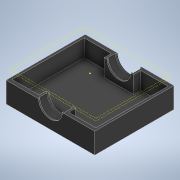
# Autodesk Inventor part: caja_base
Saved by Autodesk Inventor 2021 (Build 250183000, 183)
## iProperties
Created: 2021-12-11
Part Number: caja_base
Material: Generic
Document SubType Name: Modeling
Designer: Juan M. Casillas
Density: 1 g/cm^3
Appearance: Default
Author: Juan M. Casillas
Autodesk Inventor part; units mm, degrees
ref_plane "YZ Plane" through (0, 0, 0) normal (1, 0, 0) x (0, 1, 0)
ref_plane "XZ Plane" through (0, 0, 0) normal (0, 1, 0) x (-1, 0, 0)
ref_plane "XY Plane" through (0, 0, 0) normal (0, 0, 1) x (1, 0, 0)
sketch "Sketch1" plane through (0, 0, 0) normal (0, 1, 0) x (-1, 0, 0)
  line L0 (37.5, 32.5) -> (-37.5, 32.5)
  line L1 (-37.5, 32.5) -> (-37.5, -32.5)
  line L2 (-37.5, -32.5) -> (37.5, -32.5)
  line L3 (37.5, -32.5) -> (37.5, 32.5)
  line L4 (37.5, 32.5) -> (-37.5, -32.5) construction
  line L5 (-37.5, 32.5) -> (37.5, -32.5) construction
  line L6 (35.5, 30.5) -> (-35.5, 30.5)
  line L7 (-35.5, 30.5) -> (-35.5, -30.5)
  line L8 (-35.5, -30.5) -> (35.5, -30.5)
  line L9 (35.5, -30.5) -> (35.5, 30.5)
  line L10 (-12.5, -30.5) -> (12.5, -30.5)
  line L11 (12.5, -30.5) -> (12.5, -23.5)
  line L12 (12.5, -23.5) -> (-12.5, -23.5)
  line L13 (-12.5, -23.5) -> (-12.5, -30.5)
  line L14 (-12.5, 23.5) -> (12.5, 23.5)
  line L15 (12.5, 23.5) -> (12.5, 30.5)
  line L16 (12.5, 30.5) -> (-12.5, 30.5)
  line L17 (-12.5, 30.5) -> (-12.5, 23.5)
  point P0 (0, 0)
  point P1 (0, -30.5)
  point P2 (0, 30.5)
  point P3 (-12.5, -30.5)
  point P4 (12.5, -30.5)
  dimension "d0" = 75
  dimension "d1" = 65
  dimension "d2" = 2
  dimension "d7" = 25
  dimension "d8" = 7
  dimension "d9" = 25
  dimension "d10" = 7
  constraints: 36 end point, 8 parallel, 6 midpoint, 4 perpendicular, 3 horizontal, 3 other
  measures "d0" distance of L2.end L1.end
  measures "d1" distance of L1.end L0.end
  measures "d2" distance between parallel lines of L3 L9
  measures "d7" distance of L12.end L11.end
  measures "d8" distance of L11.end L10.end
  measures "d9" distance of L16.end L15.end
  measures "d10" distance of L15.end L14.end
extrude "Extrusion1" add sketch "Sketch1" along normal blind 20
sketch "Sketch2" plane through (0, 20, 0) normal (0, 1, 0) x (1, 0, 0)
  line L0 (-37.5, -32.5) -> (37.5, -32.5) construction
  line L1 (37.5, -32.5) -> (37.5, 32.5) construction
  line L2 (37.5, 32.5) -> (-37.5, 32.5) construction
  line L3 (-37.5, 32.5) -> (-37.5, -32.5) construction
  line L4 (-37.5, -32.5) -> (37.5, -32.5) construction
  line L5 (-35.5, -30.5) -> (-35.5, 30.5) construction
  line L6 (-35.5, 30.5) -> (35.5, 30.5) construction
  line L7 (35.5, 30.5) -> (35.5, -30.5) construction
  line L8 (35.5, -30.5) -> (-35.5, -30.5) construction
  point P0 (0, 0)
sketch "Sketch3" plane through (0, 0, 0) normal (0, -1, 0) x (1, 0, 0)
  line L0 (-37.5, 32.5) -> (37.5, 32.5) projected
  line L1 (37.5, 32.5) -> (37.5, -32.5) projected
  line L2 (37.5, -32.5) -> (-37.5, -32.5) projected
  line L3 (-37.5, -32.5) -> (-37.5, 32.5) projected
  point P0 (0, 0)
extrude "Extrusion2" add sketch "Sketch3" against normal blind 3
extrude "Extrusion3" add sketch "Sketch1" along normal blind 13 contours L15 L14 L17 L6 | L8 L13 L12 L11
sketch "Sketch4" plane through (-12.5, 3, -23.5) normal (0, 0, 1) x (1, 0, 0)
  line L0 (0, 10) -> (25, 10) construction
  point P0 (12.5, -3)
  point P1 (12.5, 10)
  constraints: 1 midpoint
hole "Hole2" at (0, 13, -23.5) direction (0, 0, -1) diameter 22 end through all both
thicken "Thicken1" operation add thickness 7 both sides no extend neighbours yes toward (0, -1, 0) faces at (36.8333, 20, 10.1667)
thicken "Thicken2" operation add thickness 7 both sides no extend neighbours yes toward (0, -1, 0) faces at (-36.8333, 20, 10.1667)
thicken "Thicken3" operation add thickness 1 both sides no extend neighbours yes toward (0, 0, 1) faces at (11.9049, 8.8371, 23.5)
thicken "Thicken4" operation add thickness 1 both sides no extend neighbours yes toward (0, 0, 1) faces at (-11.9049, 8.8371, 23.5)
thicken "Thicken5" operation add thickness 1 both sides no extend neighbours yes toward (0, 0, -1) faces at (11.9049, 8.8371, -23.5)
thicken "Thicken6" operation add thickness 1 both sides no extend neighbours yes toward (0, 0, -1) faces at (-11.9049, 8.8371, -23.5)
sketch "Sketch5" plane through (12.5, 3, 24.5) normal (0, 0, -1) x (-1, 0, 0)
  arc A0 (1.5, 10) -> (7.9174, 0) centre (12.5, 10) ccw projected
  arc A1 (17.0826, 0) -> (23.5, 10) centre (12.5, 10) ccw projected
  arc A2 (1.5, 10) -> (23.5, 10) centre (12.5, 10) ccw projected
  line L0 (1.5, 10) -> (2.5, 10)
  line L1 (23.5, 10) -> (22.5, 10)
  arc A3 (2.5, 10) -> (22.5, 10) centre (12.5, 10) ccw
  point P0 (12.5, -3)
  dimension "d39" = 1
  dimension "d40" = 1
  constraints: 4 end point, 2 horizontal, 2 point on circle, 1 centre point
  measures "d39" distance of L0.start L0.end
  measures "d40" distance of L1.start L1.end
extrude "Extrusion4" add sketch "Sketch5" against normal blind 1
thicken "Thicken7" operation add thickness 1 both sides no extend neighbours yes toward (0, 0, -1) faces at (11.5698, 8.8689, 24.5)
mirror "Mirror1" about plane through (0, 0, 0) normal (0, 0, 1) of "Extrusion4"
thicken "Thicken8" operation add thickness 1 both sides no extend neighbours yes toward (0, 0, 1) faces at (-11.5698, 8.8689, -24.5)
sketch "Sketch6" plane through (37.5, 0, -32.5) normal (0, 0, -1) x (-1, 0, 0)
  arc A0 (26.5, 13) -> (48.5, 13) centre (37.5, 13) ccw projected
  line L0 (47.5, 13) -> (48.5, 13) projected
  arc A1 (27.5, 13) -> (47.5, 13) centre (37.5, 13) ccw projected
  line L1 (26.5, 13) -> (27.5, 13) projected
  arc A2 (26.5, 13) -> (48.5, 13) centre (37.5, 13) ccw projected
  line L2 (0, 13) -> (26.5, 13) projected
  line L3 (0, 0) -> (0, 13) projected
  line L4 (0, 0) -> (75, 0) projected
  line L5 (75, 0) -> (75, 13) projected
  line L6 (48.5, 13) -> (75, 13) projected
  point P0 (37.5, 0)
extrude "Extrusion5" add sketch "Sketch6" along normal blind 1
mirror "Mirror2" about plane through (0, 0, 0) normal (0, 0, 1) of "Extrusion5"
thicken "Thicken9" operation add thickness 1 both sides no extend neighbours yes toward (0, 0, -1) faces at (-11.5698, 8.8689, -23.5)
thicken "Thicken10" operation add thickness 1 both sides no extend neighbours yes toward (0, 0, 1) faces at (11.5698, 8.8689, 23.5)
sketch "Sketch8" plane through (0, 0, 0) normal (0, -1, 0) x (1, 0, 0)
  line L0 (37.5, 33.5) -> (37.5, -33.5) projected
  line L1 (37.5, 33.5) -> (-37.5, 33.5) projected
  line L2 (-37.5, 33.5) -> (-37.5, -33.5) projected
  line L3 (37.5, -33.5) -> (-37.5, -33.5) projected
  point P0 (0, 0)
extrude "Extrusion6" add sketch "Sketch8" along normal blind 5
sketch "Sketch9" plane through (0, 3, 0) normal (0, 1, 0) x (1, 0, 0)
  line L0 (-4.5826, -24.5) -> (-4.5826, 24.5) projected
  line L1 (-4.5826, 24.5) -> (-12.5, 24.5) projected
  line L2 (-12.5, 24.5) -> (-12.5, 30.5) projected
  line L3 (-35.5, 30.5) -> (-12.5, 30.5) projected
  line L4 (-35.5, -30.5) -> (-35.5, 30.5) projected
  line L5 (-12.5, -30.5) -> (-35.5, -30.5) projected
  line L6 (-12.5, -30.5) -> (-12.5, -24.5) projected
  line L7 (-12.5, -24.5) -> (-4.5826, -24.5) projected
  line L8 (4.5826, 24.5) -> (-4.5826, 24.5) projected
  line L9 (-4.5826, -24.5) -> (-4.5826, 24.5) projected
  line L10 (-4.5826, -24.5) -> (4.5826, -24.5) projected
  line L11 (4.5826, 24.5) -> (4.5826, -24.5) projected
  line L12 (4.5826, 24.5) -> (4.5826, -24.5) projected
  line L13 (4.5826, -24.5) -> (12.5, -24.5) projected
  line L14 (12.5, -24.5) -> (12.5, -30.5) projected
  line L15 (35.5, -30.5) -> (12.5, -30.5) projected
  line L16 (35.5, 30.5) -> (35.5, -30.5) projected
  line L17 (12.5, 30.5) -> (35.5, 30.5) projected
  line L18 (12.5, 30.5) -> (12.5, 24.5) projected
  line L19 (12.5, 24.5) -> (4.5826, 24.5) projected
  line L20 (4.5826, 24.5) -> (4.5826, -24.5) projected
  line L21 (4.5826, -24.5) -> (12.5, -24.5) projected
  line L22 (12.5, -24.5) -> (12.5, -30.5) projected
  line L23 (35.5, -30.5) -> (12.5, -30.5) projected
  line L24 (35.5, 30.5) -> (35.5, -30.5) projected
  line L25 (12.5, 30.5) -> (35.5, 30.5) projected
  line L26 (12.5, 30.5) -> (12.5, 24.5) projected
  line L27 (12.5, 24.5) -> (4.5826, 24.5) projected
  point P0 (0, 0)
extrude "Extrusion7" cut sketch "Sketch9" against normal blind 5
sketch "Sketch10" plane through (0, -2, 0) normal (0, 1, 0) x (1, 0, 0)
  line L0 (12.5, -24.5) -> (-12.5, -24.5) projected
  line L1 (12.5, -30.5) -> (12.5, -24.5) projected
  line L2 (35.5, -30.5) -> (12.5, -30.5) projected
  line L3 (35.5, 30.5) -> (35.5, -30.5) projected
  line L4 (12.5, 30.5) -> (35.5, 30.5) projected
  line L5 (12.5, 24.5) -> (12.5, 30.5) projected
  line L6 (-12.5, 24.5) -> (12.5, 24.5) projected
  line L7 (-12.5, 30.5) -> (-12.5, 24.5) projected
  line L8 (-35.5, 30.5) -> (-12.5, 30.5) projected
  line L9 (-35.5, -30.5) -> (-35.5, 30.5) projected
  line L10 (-12.5, -30.5) -> (-35.5, -30.5) projected
  line L11 (-12.5, -24.5) -> (-12.5, -30.5) projected
  point P0 (0, 0)
extrude "Extrusion8" cut sketch "Sketch1" against normal blind 5 contours L9 L8 L11 L12 L13 L7 L6 L17 L14 L15
thicken "Thicken11" operation add thickness 1 both sides no extend neighbours yes toward (0, -1, 0) faces at (-4.1667, -2, 23.8333) (-4.1667, -3, 23.5)
thicken "Thicken12" operation add thickness 1 both sides no extend neighbours yes toward (0, 0, -1) faces at (4.1667, -3, -23.5)
sketch "Sketch11" plane through (0, -5, 0) normal (0, -1, 0) x (1, 0, 0)
  line L0 (12.5, -30.5) -> (12.5, -24.5) projected
  line L1 (12.5, -24.5) -> (-12.5, -24.5) projected
  line L2 (-12.5, -24.5) -> (-12.5, -30.5) projected
  line L3 (-12.5, -30.5) -> (-35.5, -30.5) projected
  line L4 (-35.5, -30.5) -> (-35.5, 30.5) projected
  line L5 (-35.5, 30.5) -> (-12.5, 30.5) projected
  line L6 (-12.5, 30.5) -> (-12.5, 24.5) projected
  line L7 (-12.5, 24.5) -> (12.5, 24.5) projected
  line L8 (12.5, 24.5) -> (12.5, 30.5) projected
  line L9 (12.5, 30.5) -> (35.5, 30.5) projected
  line L10 (35.5, 30.5) -> (35.5, -30.5) projected
  line L11 (35.5, -30.5) -> (12.5, -30.5) projected
  line L12 (-37.5, -33.5) -> (37.5, -33.5) projected
  line L13 (37.5, -33.5) -> (37.5, 33.5) projected
  line L14 (37.5, 33.5) -> (-37.5, 33.5) projected
  line L15 (-37.5, 33.5) -> (-37.5, -33.5) projected
  point P0 (0, 0)
extrude "Extrusion9" cut sketch "Sketch11" against normal blind 3.46 contours L0 L1 L2 L3 L4 L5 L6 L7 L8 L9 L10 L11 | L15 L14 L13 L12
sketch "Sketch12" plane through (0, -1.54, 0) normal (0, -1, 0) x (1, 0, 0)
  line L0 (12.5, -24.5) -> (12.5, -30.5) construction
  line L1 (-12.5, -24.5) -> (12.5, -24.5) construction
  line L2 (-12.5, -30.5) -> (-12.5, -24.5) construction
  line L3 (-35.5, -30.5) -> (-12.5, -30.5) construction
  line L4 (-35.5, 30.5) -> (-35.5, -30.5) construction
  line L5 (-12.5, 30.5) -> (-35.5, 30.5) construction
  line L6 (-12.5, 24.5) -> (-12.5, 30.5) construction
  line L7 (12.5, 24.5) -> (-12.5, 24.5) construction
  line L8 (12.5, 30.5) -> (12.5, 24.5) construction
  line L9 (35.5, 30.5) -> (12.5, 30.5) construction
  line L10 (35.5, -30.5) -> (35.5, 30.5) construction
  line L11 (12.5, -30.5) -> (35.5, -30.5) construction
  line L12 (37.5, 33.5) -> (37.5, -33.5) construction
  line L13 (-37.5, 33.5) -> (37.5, 33.5) construction
  line L14 (-37.5, -33.5) -> (-37.5, 33.5) construction
  line L15 (37.5, -33.5) -> (-37.5, -33.5) construction
  line L16 (37.5, -33.5) -> (-37.5, -33.5)
  line L17 (-37.5, -33.5) -> (-37.5, 33.5)
  line L18 (-37.5, 33.5) -> (37.5, 33.5)
  line L19 (37.5, 33.5) -> (37.5, -33.5)
  point P0 (0, 0)
  constraints: 8 end point, 2 parallel, 1 horizontal, 1 perpendicular
extrude "Extrusion10" add sketch "Sketch12" along normal blind 3
body "Solid1"
